Xiaoyu Qi-LED Case-Lid (Used) (Autodesk Fusion 360 design; units mm, degrees)
Autodesk Fusion 360 part; units mm, degrees
sketch "Sketch1" plane through (0, 0, 0) normal (0, 1, 0) x (1, 0, 0)
  line L0 (47, 36) -> (-47, 36)
  line L1 (-47, 36) -> (-47, -36)
  line L2 (-47, -36) -> (47, -36)
  line L3 (47, -36) -> (47, 36)
  line L4 (47, 36) -> (-47, -36) construction
  line L5 (-47, 36) -> (47, -36) construction
  dimension "d1" = 72
  dimension "d2" = 94
  measures "d1" distance of L0.end L1.end
  measures "d2" distance of L0.start L0.end
extrude "Extrude1" add sketch "Sketch1" along normal blind 5
sketch "Sketch2" plane through (0, 5, 0) normal (0, 1, 0) x (-1, 0, 0)
  line L0 (-47, 36) -> (-47, -36)
  line L1 (-47, -36) -> (47, -36)
  line L2 (47, -36) -> (47, 36)
  line L3 (47, 36) -> (-47, 36)
  line L4 (-41.6, -30.6) -> (41.6, -30.6)
  line L5 (41.6, -30.6) -> (41.6, 30.6)
  line L6 (41.6, 30.6) -> (-41.6, 30.6)
  line L7 (-41.6, 30.6) -> (-41.6, -30.6)
  line L8 (-41.6, -30.6) -> (41.6, 30.6) construction
  line L9 (41.6, -30.6) -> (-41.6, 30.6) construction
  dimension "d5" = 83.2
  dimension "d6" = 61.2
  measures "d5" distance of L5.end L6.end
  measures "d6" distance of L4.start L6.end
extrude "Extrude2" add sketch "Sketch2" along normal blind 9.8 contours L4 L5 L6 L7
fillet "Fillet1" radius 2 4 edges at (47, 2.5, -36) (47, 2.5, 36) (-47, 2.5, 36) (-47, 2.5, -36)
fillet "Fillet2" radius 2 8 edges at (0, 0, -36) (-46.4142, 0, -35.4142) (-47, 0, 0) (-46.4142, 0, 35.4142) (0, 0, 36) (46.4142, 0, 35.4142) (47, 0, 0) (46.4142, 0, -35.4142)
sketch "Sketch3" plane through (0, 14.8, 0) normal (0, 1, 0) x (-1, 0, 0)
  line L0 (-41.6, 30.6) -> (-41.6, -30.6)
  line L1 (-41.6, -30.6) -> (41.6, -30.6)
  line L2 (41.6, -30.6) -> (41.6, 30.6)
  line L3 (41.6, 30.6) -> (-41.6, 30.6)
  line L4 (-38.6, -28) -> (38.6, -28)
  line L5 (38.6, -28) -> (38.6, 28)
  line L6 (38.6, 28) -> (-38.6, 28)
  line L7 (-38.6, 28) -> (-38.6, -28)
  line L8 (-38.6, -28) -> (38.6, 28) construction
  line L9 (38.6, -28) -> (-38.6, 28) construction
  line L10 (-45, -34) -> (45, -34)
  dimension "d11" = 56
  dimension "d12" = 77.2
  dimension "d13" = 90
  measures "d11" distance of L4.start L6.end
  measures "d12" distance of L5.end L6.end
  measures "d13" distance of L10.start L10.end
extrude "Extrude3" cut sketch "Sketch3" against normal blind 9.8 contours L4 L5 L6 L7
sketch "Sketch4" plane through (0, 0, -30.6) normal (0, 0, -1) x (-1, 0, 0)
  line L0 (-41.6, 5) -> (41.6, 5)
  line L1 (41.6, 5) -> (41.6, 14.8)
  line L2 (41.6, 14.8) -> (-41.6, 14.8)
  line L3 (-41.6, 14.8) -> (-41.6, 5)
  line L4 (10, 14) -> (-10, 14)
  line L5 (-10, 14) -> (-10, 12)
  line L6 (-10, 12) -> (10, 12)
  line L7 (10, 12) -> (10, 14)
  line L8 (10, 14) -> (-10, 12) construction
  line L9 (-10, 14) -> (10, 12) construction
  point P0 (0, 13)
  dimension "d16" = 20
  dimension "d17" = 2
  measures "d16" distance of L4.start L4.end
  measures "d17" distance of L4.start L6.end
extrude "Extrude4" add sketch "Sketch4" along normal blind 1.2 contours L4 L5 L6 L7
sketch "Sketch5" plane through (10, 0, 0) normal (1, 0, 0) x (0, 0, -1)
  line L0 (30.6, 14) -> (30.6, 12)
  line L1 (30.6, 12) -> (31.8, 12)
  line L2 (31.8, 12) -> (31.8, 14)
  line L3 (31.8, 14) -> (30.6, 14)
  point P0 (31.8, 14)
  point P1 (31.8, 12)
  point P2 (31.8, 12)
  point P3 (31.8, 12)
  point P4 (31.8, 12)
  point P5 (31.8, 12)
  point P6 (31.8, 14)
  point P7 (31.8, 14)
  point P8 (31.8, 14)
  point P9 (31.8, 14)
  point P10 (31.8, 14)
  point P11 (31.8, 14)
  point P12 (31.8, 14)
  point P13 (31.8, 14)
  point P14 (31.8, 14)
  point P15 (31.8, 14)
  point P16 (31.8, 12)
  point P17 (31.8, 14)
  point P18 (31.8, 12)
  point P19 (31.8, 14)
ref_plane "WorkPlane2" through (0, 9.9, 0) normal (0, 0, 1) x (-1, 0, 0)
ref_plane "WorkPlane1" through (0, 9.9, 30.6) normal (0, 0, 1) x (1, 0, 0)
ref_plane "WorkPlane3" through (0, 13, -26.8) normal (0, 0, -1) x (-1, 0, 0)
ref_plane "WorkPlane4" through (0, 13, -26.8) normal (0, 0, -1) x (-1, 0, 0)
mirror "Mirror1" about plane through (0, 9.9, 0) normal (0, 0, 1) of "Extrude4"
chamfer "Chamfer1" distance 1 angle 45 2 edges at (0, 14, 31.8) (0, 12, 31.8)
chamfer "Chamfer2" distance 1 angle 45 2 edges at (0, 14, -31.8) (0, 12, -31.8)
sketch "Sketch6" plane through (0, 14.8, 0) normal (0, 1, 0) x (-1, 0, 0)
  line L0 (38.6, -28) -> (-38.6, -28)
  line L1 (-38.6, -28) -> (-38.6, 28)
  line L2 (-38.6, 28) -> (38.6, 28)
  line L3 (38.6, 28) -> (38.6, -28)
  line L4 (-41.6, 30.6) -> (-41.6, -30.6)
  line L5 (-41.6, -30.6) -> (41.6, -30.6)
  line L6 (41.6, -30.6) -> (41.6, 30.6)
  line L7 (41.6, 30.6) -> (-41.6, 30.6)
  point P0 (42.1144, 28)
  point P1 (-41.6, 30.6)
sketch "Sketch7" plane through (0, 5, 0) normal (0, 1, 0) x (-1, 0, 0)
  arc A0 (45, -36) -> (47, -34) centre (45, -34) ccw
  line L0 (47, -34) -> (47, 34)
  arc A1 (47, 34) -> (45, 36) centre (45, 34) ccw
  line L1 (45, 36) -> (-45, 36)
  arc A2 (-45, 36) -> (-47, 34) centre (-45, 34) ccw
  line L2 (-47, 34) -> (-47, -34)
  arc A3 (-47, -34) -> (-45, -36) centre (-45, -34) ccw
  line L3 (-45, -36) -> (45, -36)
  line L4 (-41.6, 30.6) -> (41.6, 30.6)
  line L5 (41.6, 30.6) -> (41.6, -30.6)
  line L6 (41.6, -30.6) -> (-41.6, -30.6)
  line L7 (-41.6, -30.6) -> (-41.6, 30.6)
  line L8 (45, -34) -> (-45, -34)
  line L9 (-45, -34) -> (-45, 34)
  line L10 (-45, 34) -> (45, 34)
  line L11 (45, 34) -> (45, -34)
extrude "Extrude5" cut sketch "Sketch7" against normal blind 5 contours A0 L0 A1 L1 A2 L2 A3 L3
fillet "Fillet3" radius 2 8 edges at (-45, 2.5, -34) (0, 0, -34) (-45, 0, 0) (45, 2.5, -34) (45, 0, 0) (45, 2.5, 34) (0, 0, 34) (-45, 2.5, 34)
